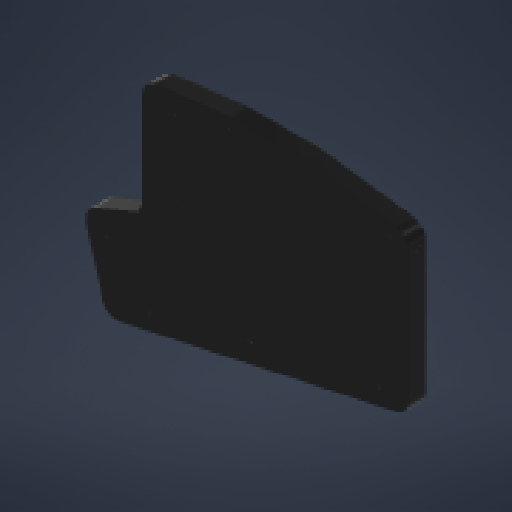
# Autodesk Inventor part: Case Bottom
Saved by Autodesk Inventor 2024.3 (Build 283343000, 343)
## iProperties
Created: 2024-12-13
Part Number: Case Bottom
Material: Generic
Document SubType Name: Modeling
Designer: micha
Density: 1 g/cm^3
Appearance: Smooth - Black
Author: micha
Autodesk Inventor part; units mm, degrees
ref_plane "YZ Plane" through (0, 0, 0) normal (1, 0, 0) x (0, 1, 0)
ref_plane "XZ Plane" through (0, 0, 0) normal (0, 1, 0) x (-1, 0, 0)
ref_plane "XY Plane" through (0, 0, 0) normal (0, 0, 1) x (1, 0, 0)
sketch "Sketch1" plane through (0, 0, 0) normal (0, 0, 1) x (1, 0, 0)
  arc A0 (-212.538998, -59.46938) -> (-218.504473, -64.85881) centre (-212.540124, -65.464394) ccw
  line L0 (-174.03635, -54.760868) -> (-212.538998, -59.46938)
  arc A1 (-171.723941, -54.62) -> (-174.03635, -54.760868) centre (-171.723929, -73.670234) ccw
  line L1 (-134.883154, -54.62) -> (-171.723941, -54.62)
  arc A2 (-132.280238, -54.798664) -> (-134.883154, -54.62) centre (-134.883228, -73.671057) ccw
  line L2 (-83.542158, -61.521089) -> (-132.280238, -54.798664)
  arc A3 (-79.229999, -66.473551) -> (-83.542158, -61.521089) centre (-84.229999, -66.47355) ccw
  line L3 (-79.477279, -138.022361) -> (-79.229999, -66.473551)
  arc A4 (-82.987736, -142.795333) -> (-79.477279, -138.022361) centre (-84.477328, -138.022325) ccw
  line L4 (-234.360737, -175.723727) -> (-82.987736, -142.795333)
  arc A5 (-240.233758, -172.877296) -> (-234.360737, -175.723727) centre (-235.745406, -171.098608) ccw
  line L5 (-249.32837, -140.9769) -> (-240.233758, -172.877296)
  arc A6 (-246.255809, -134.396385) -> (-249.32837, -140.9769) centre (-243.556977, -139.664093) ccw
  line L6 (-224.253241, -125.409604) -> (-246.255809, -134.396385)
  arc A7 (-224.253241, -125.409604) -> (-221.422813, -123.130228) centre (-226.654291, -119.531049) ccw
  line L7 (-220.681757, -122.053089) -> (-221.422813, -123.130228)
  arc A8 (-220.681757, -122.053089) -> (-218.444728, -114.839545) centre (-231.14451, -114.854791) ccw
  line L8 (-218.504474, -64.85881) -> (-218.444728, -114.839545)
  circle A9 centre (-163.195, -152.4) radius 1.05
  circle A10 centre (-92.075, -138.43) radius 1.05
  circle A11 centre (-86.11, -127.04) radius 0.8509
  circle A12 centre (-91.61, -127.04) radius 1.7145
  circle A13 centre (-97.11, -127.04) radius 0.8509
  circle A14 centre (-104.11, -127.04) radius 0.8509
  circle A15 centre (-122.11, -139.04) radius 0.8509
  circle A16 centre (-122.61, -135.29) radius 1.5
  circle A17 centre (-109.61, -127.04) radius 1.7145
  circle A18 centre (-115.11, -127.04) radius 0.8509
  circle A19 centre (-86.61, -123.29) radius 1.5
  circle A20 centre (-91.61, -121.09) radius 1.5
  circle A21 centre (-96.61, -123.29) radius 1.5
  circle A22 centre (-104.61, -123.29) radius 1.5
  circle A23 centre (-109.61, -121.09) radius 1.5
  circle A24 centre (-114.61, -123.29) radius 1.5
  circle A25 centre (-122.11, -122.04) radius 0.8509
  circle A26 centre (-122.61, -118.29) radius 1.5
  circle A27 centre (-127.61, -139.04) radius 1.7145
  circle A28 centre (-133.11, -139.04) radius 0.8509
  circle A29 centre (-132.61, -135.29) radius 1.5
  circle A30 centre (-140.11, -136.54) radius 0.8509
  circle A31 centre (-127.61, -133.09) radius 1.5
  circle A32 centre (-140.61, -132.79) radius 1.5
  circle A33 centre (-145.61, -136.54) radius 1.7145
  circle A34 centre (-151.11, -136.54) radius 0.8509
  circle A35 centre (-158.11, -139.04) radius 0.8509
  circle A36 centre (-163.61, -139.04) radius 1.7145
  circle A37 centre (-158.61, -135.29) radius 1.5
  circle A38 centre (-145.61, -130.59) radius 1.5
  circle A39 centre (-150.61, -132.79) radius 1.5
  circle A40 centre (-163.61, -133.09) radius 1.5
  circle A41 centre (-127.61, -122.04) radius 1.7145
  circle A42 centre (-133.11, -122.04) radius 0.8509
  circle A43 centre (-140.11, -119.54) radius 0.8509
  circle A44 centre (-127.61, -116.09) radius 1.5
  circle A45 centre (-132.61, -118.29) radius 1.5
  circle A46 centre (-140.61, -115.79) radius 1.5
  circle A47 centre (-145.61, -119.54) radius 1.7145
  circle A48 centre (-151.11, -119.54) radius 0.8509
  circle A49 centre (-158.11, -122.04) radius 0.8509
  circle A50 centre (-163.61, -122.04) radius 1.7145
  circle A51 centre (-145.61, -113.59) radius 1.5
  circle A52 centre (-150.61, -115.79) radius 1.5
  circle A53 centre (-158.61, -118.29) radius 1.5
  circle A54 centre (-163.61, -116.09) radius 1.5
  circle A55 centre (-198.250758, -148.049295) radius 0.8509
  circle A56 centre (-187.91414, -144.287073) radius 0.8509
  circle A57 centre (-193.082449, -146.168184) radius 1.7145
  circle A58 centre (-189.666561, -140.934236) radius 1.5
  circle A59 centre (-199.063488, -144.354437) radius 1.5
  circle A60 centre (-195.117469, -140.577013) radius 1.5
  circle A61 centre (-217.896589, -166.960904) radius 1.05
  circle A62 centre (-217.279534, -154.975203) radius 0.8509
  circle A63 centre (-236.308309, -161.901111) radius 0.8509
  circle A64 centre (-225.971691, -158.138889) radius 0.8509
  circle A65 centre (-231.14, -160.02) radius 1.7145
  circle A66 centre (-227.724112, -154.786052) radius 1.5
  circle A67 centre (-237.121039, -158.206253) radius 1.5
  circle A68 centre (-233.17502, -154.428829) radius 1.5
  circle A69 centre (-206.942916, -151.212981) radius 0.8509
  circle A70 centre (-212.111225, -153.094092) radius 1.7145
  circle A71 centre (-208.695337, -147.860144) radius 1.5
  circle A72 centre (-218.092264, -151.280345) radius 1.5
  circle A73 centre (-214.146245, -147.502921) radius 1.5
  circle A74 centre (-241.3, -142.24) radius 1.05
  circle A75 centre (-169.11, -139.04) radius 0.8509
  circle A76 centre (-168.61, -135.29) radius 1.5
  circle A77 centre (-201.862915, -128.352981) radius 0.8509
  circle A78 centre (-169.11, -122.04) radius 0.8509
  circle A79 centre (-176.11, -124.54) radius 0.8509
  circle A80 centre (-181.61, -124.54) radius 1.7145
  circle A81 centre (-176.61, -120.79) radius 1.5
  circle A82 centre (-168.61, -118.29) radius 1.5
  circle A83 centre (-181.61, -118.59) radius 1.5
  circle A84 centre (-187.11, -124.54) radius 0.8509
  circle A85 centre (-186.61, -120.79) radius 1.5
  circle A86 centre (-194.500629, -125.059163) radius 0.4
  circle A87 centre (-194.500629, -123.059163) radius 0.381
  circle A88 centre (-194.500629, -121.059163) radius 0.381
  circle A89 centre (-201.350629, -114.209163) radius 0.4
  circle A90 centre (-220.891691, -135.278889) radius 0.8509
  circle A91 centre (-207.031224, -130.234092) radius 1.7145
  circle A92 centre (-212.199533, -132.115203) radius 0.8509
  circle A93 centre (-222.644112, -131.926052) radius 1.5
  circle A94 centre (-213.012263, -128.420345) radius 1.5
  circle A95 centre (-226.06, -137.16) radius 1.7145
  circle A96 centre (-231.228309, -139.041111) radius 0.8509
  circle A97 centre (-232.041039, -135.346253) radius 1.5
  circle A98 centre (-228.09502, -131.568829) radius 1.5
  circle A99 centre (-203.615336, -125.000144) radius 1.5
  circle A100 centre (-209.066244, -124.642921) radius 1.5
  circle A101 centre (-203.350629, -114.209163) radius 0.4
  circle A102 centre (-205.350629, -114.209163) radius 0.4
  circle A103 centre (-86.11, -110.04) radius 0.8509
  circle A104 centre (-91.61, -110.04) radius 1.7145
  circle A105 centre (-86.61, -106.29) radius 1.5
  circle A106 centre (-97.11, -110.04) radius 0.8509
  circle A107 centre (-104.11, -110.04) radius 0.8509
  circle A108 centre (-96.61, -106.29) radius 1.5
  circle A109 centre (-104.61, -106.29) radius 1.5
  circle A110 centre (-91.61, -104.09) radius 1.5
  circle A111 centre (-109.61, -110.04) radius 1.7145
  circle A112 centre (-115.11, -110.04) radius 0.8509
  circle A113 centre (-114.61, -106.29) radius 1.5
  circle A114 centre (-109.61, -104.09) radius 1.5
  circle A115 centre (-122.11, -105.04) radius 0.8509
  circle A116 centre (-122.61, -101.29) radius 1.5
  circle A117 centre (-86.11, -93.04) radius 0.8509
  circle A118 centre (-91.61, -93.04) radius 1.7145
  circle A119 centre (-97.11, -93.04) radius 0.8509
  circle A120 centre (-104.11, -93.04) radius 0.8509
  circle A121 centre (-86.61, -89.29) radius 1.5
  circle A122 centre (-91.61, -87.09) radius 1.5
  circle A123 centre (-96.61, -89.29) radius 1.5
  circle A124 centre (-104.61, -89.29) radius 1.5
  circle A125 centre (-109.61, -93.04) radius 1.7145
  circle A126 centre (-115.11, -93.04) radius 0.8509
  circle A127 centre (-109.61, -87.09) radius 1.5
  circle A128 centre (-114.61, -89.29) radius 1.5
  circle A129 centre (-122.11, -88.04) radius 0.8509
  circle A130 centre (-127.61, -105.04) radius 1.7145
  circle A131 centre (-133.11, -105.04) radius 0.8509
  circle A132 centre (-127.61, -99.09) radius 1.5
  circle A133 centre (-132.61, -101.29) radius 1.5
  circle A134 centre (-140.11, -102.54) radius 0.8509
  circle A135 centre (-140.61, -98.79) radius 1.5
  circle A136 centre (-145.61, -102.54) radius 1.7145
  circle A137 centre (-151.11, -102.54) radius 0.8509
  circle A138 centre (-150.61, -98.79) radius 1.5
  circle A139 centre (-158.11, -105.04) radius 0.8509
  circle A140 centre (-163.61, -105.04) radius 1.7145
  circle A141 centre (-158.61, -101.29) radius 1.5
  circle A142 centre (-163.61, -99.09) radius 1.5
  circle A143 centre (-127.61, -88.04) radius 1.7145
  circle A144 centre (-133.11, -88.04) radius 0.8509
  circle A145 centre (-140.11, -85.54) radius 0.8509
  circle A146 centre (-145.61, -96.59) radius 1.5
  circle A147 centre (-145.61, -85.54) radius 1.7145
  circle A148 centre (-151.11, -85.54) radius 0.8509
  circle A149 centre (-158.11, -88.04) radius 0.8509
  circle A150 centre (-163.61, -88.04) radius 1.7145
  circle A151 centre (-86.11, -76.04) radius 0.8509
  circle A152 centre (-91.61, -76.04) radius 1.7145
  circle A153 centre (-86.61, -72.29) radius 1.5
  circle A154 centre (-97.11, -76.04) radius 0.8509
  circle A155 centre (-104.11, -76.04) radius 0.8509
  circle A156 centre (-96.61, -72.29) radius 1.5
  circle A157 centre (-104.61, -72.29) radius 1.5
  circle A158 centre (-122.61, -84.29) radius 1.5
  circle A159 centre (-109.61, -76.04) radius 1.7145
  circle A160 centre (-115.11, -76.04) radius 0.8509
  circle A161 centre (-114.61, -72.29) radius 1.5
  circle A162 centre (-122.11, -71.04) radius 0.8509
  circle A163 centre (-91.61, -70.09) radius 1.5
  circle A164 centre (-86.119409, -65.103368) radius 1.05
  circle A165 centre (-109.61, -70.09) radius 1.5
  circle A166 centre (-122.61, -67.29) radius 1.5
  circle A167 centre (-127.61, -82.09) radius 1.5
  circle A168 centre (-132.61, -84.29) radius 1.5
  circle A169 centre (-140.61, -81.79) radius 1.5
  circle A170 centre (-127.61, -71.04) radius 1.7145
  circle A171 centre (-133.11, -71.04) radius 0.8509
  circle A172 centre (-150.61, -81.79) radius 1.5
  circle A173 centre (-145.61, -79.59) radius 1.5
  circle A174 centre (-158.61, -84.29) radius 1.5
  circle A175 centre (-163.61, -82.09) radius 1.5
  circle A176 centre (-158.11, -71.04) radius 0.8509
  circle A177 centre (-163.61, -71.04) radius 1.7145
  circle A178 centre (-127.61, -65.09) radius 1.5
  circle A179 centre (-132.61, -67.29) radius 1.5
  circle A180 centre (-140.11, -68.54) radius 0.8509
  circle A181 centre (-140.61, -64.79) radius 1.5
  circle A182 centre (-145.61, -68.54) radius 1.7145
  circle A183 centre (-151.11, -68.54) radius 0.8509
  circle A184 centre (-150.61, -64.79) radius 1.5
  circle A185 centre (-158.61, -67.29) radius 1.5
  circle A186 centre (-163.61, -65.09) radius 1.5
  circle A187 centre (-145.61, -62.59) radius 1.5
  circle A188 centre (-176.11, -107.54) radius 0.8509
  circle A189 centre (-181.61, -107.54) radius 1.7145
  circle A190 centre (-169.11, -105.04) radius 0.8509
  circle A191 centre (-168.61, -101.29) radius 1.5
  circle A192 centre (-176.61, -103.79) radius 1.5
  circle A193 centre (-181.61, -101.59) radius 1.5
  circle A194 centre (-187.11, -107.54) radius 0.8509
  circle A195 centre (-202.046541, -105.604357) radius 1.05
  circle A196 centre (-186.61, -103.79) radius 1.5
  circle A197 centre (-169.11, -88.04) radius 0.8509
  circle A198 centre (-176.11, -90.54) radius 0.8509
  circle A199 centre (-181.61, -90.54) radius 1.7145
  circle A200 centre (-176.61, -86.79) radius 1.5
  circle A201 centre (-195.58, -92.956268) radius 0.5461
  circle A202 centre (-187.11, -90.54) radius 0.8509
  circle A203 centre (-186.61, -86.79) radius 1.5
  circle A204 centre (-195.58, -90.416268) radius 0.5461
  circle A205 centre (-195.58, -87.876268) radius 0.5461
  circle A206 centre (-195.58, -85.336268) radius 0.5461
  arc A207 (-207.555848, -104.429405) -> (-207.555848, -103.529405) centre (-207.555848, -103.979405) ccw
  line L9 (-207.555848, -103.529405) -> (-208.155848, -103.529405)
  arc A208 (-208.155848, -103.529405) -> (-208.155848, -104.429405) centre (-208.155848, -103.979405) ccw
  line L10 (-208.155848, -104.429405) -> (-207.555848, -104.429405)
  arc A209 (-211.555848, -104.429405) -> (-211.555848, -103.529405) centre (-211.555848, -103.979405) ccw
  line L11 (-211.555848, -103.529405) -> (-212.155848, -103.529405)
  arc A210 (-212.155848, -103.529405) -> (-212.155848, -104.429405) centre (-212.155848, -103.979405) ccw
  line L12 (-212.155848, -104.429405) -> (-211.555848, -104.429405)
  arc A211 (-206.455848, -102.129405) -> (-206.455848, -101.229405) centre (-206.455848, -101.679405) ccw
  line L13 (-206.455848, -101.229405) -> (-207.055848, -101.229405)
  arc A212 (-207.055848, -101.229405) -> (-207.055848, -102.129405) centre (-207.055848, -101.679405) ccw
  line L14 (-207.055848, -102.129405) -> (-206.455848, -102.129405)
  arc A213 (-206.455848, -99.829405) -> (-206.455848, -98.929405) centre (-206.455848, -99.379405) ccw
  line L15 (-206.455848, -98.929405) -> (-207.055848, -98.929405)
  arc A214 (-207.055848, -98.929405) -> (-207.055848, -99.829405) centre (-207.055848, -99.379405) ccw
  line L16 (-207.055848, -99.829405) -> (-206.455848, -99.829405)
  circle A215 centre (-209.455848, -101.679405) radius 0.75
  circle A216 centre (-209.455848, -99.379405) radius 0.75
  arc A217 (-214.555848, -104.429405) -> (-214.555848, -103.529405) centre (-214.555848, -103.979405) ccw
  line L17 (-214.555848, -103.529405) -> (-215.155848, -103.529405)
  arc A218 (-215.155848, -103.529405) -> (-215.155848, -104.429405) centre (-215.155848, -103.979405) ccw
  line L18 (-215.155848, -104.429405) -> (-214.555848, -104.429405)
  circle A219 centre (-216.455848, -101.679405) radius 0.75
  circle A220 centre (-216.455848, -99.379405) radius 0.75
  arc A221 (-207.555848, -97.529405) -> (-207.555848, -96.629405) centre (-207.555848, -97.079405) ccw
  line L19 (-207.555848, -96.629405) -> (-208.155848, -96.629405)
  arc A222 (-208.155848, -96.629405) -> (-208.155848, -97.529405) centre (-208.155848, -97.079405) ccw
  line L20 (-208.155848, -97.529405) -> (-207.555848, -97.529405)
  arc A223 (-211.555848, -97.529405) -> (-211.555848, -96.629405) centre (-211.555848, -97.079405) ccw
  line L21 (-211.555848, -96.629405) -> (-212.155848, -96.629405)
  arc A224 (-212.155848, -96.629405) -> (-212.155848, -97.529405) centre (-212.155848, -97.079405) ccw
  line L22 (-212.155848, -97.529405) -> (-211.555848, -97.529405)
  circle A225 centre (-210.82, -92.956268) radius 0.5461
  arc A226 (-214.555848, -97.529405) -> (-214.555848, -96.629405) centre (-214.555848, -97.079405) ccw
  line L23 (-214.555848, -96.629405) -> (-215.155848, -96.629405)
  arc A227 (-215.155848, -96.629405) -> (-215.155848, -97.529405) centre (-215.155848, -97.079405) ccw
  line L24 (-215.155848, -97.529405) -> (-214.555848, -97.529405)
  circle A228 centre (-210.82, -90.416268) radius 0.5461
  circle A229 centre (-210.82, -87.876268) radius 0.5461
  circle A230 centre (-210.82, -85.336268) radius 0.5461
  circle A231 centre (-168.61, -84.29) radius 1.5
  circle A232 centre (-181.61, -84.59) radius 1.5
  circle A233 centre (-169.11, -71.04) radius 0.8509
  circle A234 centre (-176.11, -73.54) radius 0.8509
  circle A235 centre (-181.61, -73.54) radius 1.7145
  circle A236 centre (-195.58, -82.796268) radius 0.5461
  circle A237 centre (-195.58, -80.256268) radius 0.5461
  circle A238 centre (-187.11, -73.54) radius 0.8509
  circle A239 centre (-195.58, -77.716268) radius 0.5461
  circle A240 centre (-195.58, -75.176268) radius 0.5461
  circle A241 centre (-199.5, -77.736268) radius 0.2
  circle A242 centre (-199.45, -75.286268) radius 0.2
  circle A243 centre (-195.58, -72.636268) radius 0.5461
  circle A244 centre (-199.45, -72.636268) radius 0.2
  circle A245 centre (-168.61, -67.29) radius 1.5
  circle A246 centre (-176.61, -69.79) radius 1.5
  circle A247 centre (-181.61, -67.59) radius 1.5
  circle A248 centre (-174.342576, -58.074257) radius 1.05
  circle A249 centre (-186.61, -69.79) radius 1.5
  circle A250 centre (-195.58, -70.096268) radius 0.5461
  circle A251 centre (-195.58, -67.556268) radius 0.5461
  circle A252 centre (-199.486417, -69.986269) radius 0.2
  circle A253 centre (-195.58, -65.016268) radius 0.5461
  circle A254 centre (-210.82, -82.796268) radius 0.5461
  circle A255 centre (-210.82, -80.256268) radius 0.5461
  circle A256 centre (-206.55, -77.786268) radius 0.2
  circle A257 centre (-206.55, -75.236268) radius 0.2
  circle A258 centre (-210.82, -77.716268) radius 0.5461
  circle A259 centre (-210.82, -75.176268) radius 0.5461
  circle A260 centre (-206.55, -72.636268) radius 0.2
  circle A261 centre (-210.82, -72.636268) radius 0.5461
  circle A262 centre (-206.55, -70.186268) radius 0.2
  circle A263 centre (-210.82, -70.096268) radius 0.5461
  circle A264 centre (-210.82, -67.556268) radius 0.5461
  circle A265 centre (-204.203785, -64.736757) radius 1.05
  circle A266 centre (-210.82, -65.016268) radius 0.5461
  arc A267 (-212.752532, -56.29684) -> (-221.663233, -64.538089) centre (-212.540124, -65.464394) ccw
  line L25 (-212.752532, -56.29684) -> (-174.421768, -51.609348)
  arc A268 (-171.723929, -51.445) -> (-174.421768, -51.609348) centre (-171.723929, -73.670234) ccw
  line L26 (-171.723929, -51.445) -> (-134.883228, -51.445)
  arc A269 (-131.846348, -51.653451) -> (-134.883228, -51.445) centre (-134.883228, -73.671057) ccw
  line L27 (-131.846348, -51.653451) -> (-83.113, -58.375223)
  arc A270 (-76.055001, -66.479709) -> (-83.113, -58.375223) centre (-84.229999, -66.47355) ccw
  line L28 (-76.055001, -66.479709) -> (-76.302281, -138.028529)
  arc A271 (-82.192563, -145.87161) -> (-76.302281, -138.028529) centre (-84.477328, -138.022325) ccw
  line L29 (-82.192563, -145.87161) -> (-233.581807, -178.803537)
  arc A272 (-243.249182, -173.880774) -> (-233.581807, -178.803537) centre (-235.745406, -171.098608) ccw
  line L30 (-243.249182, -173.880774) -> (-252.402726, -141.773666)
  arc A273 (-247.568867, -131.503069) -> (-252.402726, -141.773666) centre (-243.556977, -139.664093) ccw
  line L31 (-247.568867, -131.503069) -> (-225.453766, -122.470324)
  arc A274 (-225.453766, -122.470324) -> (-224.038554, -121.330638) centre (-226.654291, -119.531049) ccw
  line L32 (-224.038554, -121.330638) -> (-223.297462, -120.253446)
  arc A275 (-223.297462, -120.253446) -> (-221.619726, -114.843405) centre (-231.14451, -114.854791) ccw
  line L33 (-221.619726, -114.843405) -> (-221.663233, -78.447127)
  line L34 (-221.663233, -78.447127) -> (-221.663233, -64.538089)
  point P0 (0, 0)
  point P1 (-218.504473, -64.85881)
  dimension "d0" = 3.175
  constraints: 20 end point, 18 point on circle, 9 centre point, 1 vertical, 17 other
  measures "d0" distance between parallel lines of L3 L28
extrude "Extrusion1" add sketch "Sketch1" along normal blind 3.175 contours L0 A1 L1 A2 L2 A3 L3 A4 L4 A5 L5 A6 L6 A7 L7 A8 L8 A0 | A11 | A12 | A13 | A14 | A15 | A16 | A17 | A18 | A19 | A20 | A21 | A22 | A23 | A24 | A25 | A26 | A27 | A28 | A29 | A30 | A31 | A32 | A33 | A34 | A35 | A36 | A37 | A38 | A39 | A40 | A41 | A42 | A43 | A44 | A45 | A46 | A47 | A48 | A49 | A50 | A51 | A52 | A53 | A54 | A55 | A56 | A57 | A58 | A59 | A60 | A62 | A63 | A64 | A65 | A66 | A67 | A68 | A69 | A70 | A71 | A72 | A73 | A75 | A76 | A77 | A78 | A79 | A80 | A81 | A82 | A83 | A84 | A85 | A86 | A87 | A88 | A89 | A90 | A91 | A92 | A93 | A94 | A95 | A96 | A97 | A98 | A99 | A100 | A101 | A102 | A103 | A104 | A105 | A106 | A107 | A108 | A109 | A110 | A111 | A112 | A113 | A114 | A115 | A116 | A117 | A118 | A119 | A120 | A121 | A122 | A123 | A124 | A125 | A126 | A127 | A128 | A129 | A130 | A131 | A132 | A133 | A134 | A135 | A136 | A137 | A138 | A139 | A140 | A141 | A142 | A143 | A144 | A145 | A146 | A147 | A148 | A149 | A150 | A151 | A152 | A153 | A154 | A155 | A156 | A157 | A158 | A159 | A160 | A161 | A162 | A163 | A165 | A166 | A167 | A168 | A169 | A170 | A171 | A172 | A173 | A174 | A175 | A176 | A177 | A178 | A179 | A180 | A181 | A182 | A183 | A184 | A185 | A186 | A187 | A188 | A189 | A190 | A191 | A192 | A193 | A194 | A196 | A197 | A198 | A199 | A200 | A201 | A202 | A203 | A204 | A205 | A206 | L10 A208 L9 A207 | L12 A210 L11 A209 | L14 A212 L13 A211 | L16 A214 L15 A213 | A215 | A216 | L18 A218 L17 A217 | A219 | A220 | L20 A222 L19 A221 | L22 A224 L21 A223 | A225 | L24 A227 L23 A226 | A228 | A229 | A230 | A231 | A232 | A233 | A234 | A235 | A236 | A237 | A238 | A239 | A240 | A241 | A242 | A243 | A244 | A245 | A246 | A247 | A249 | A250 | A251 | A252 | A253 | A254 | A255 | A256 | A257 | A258 | A259 | A260 | A261 | A262 | A263 | A264 | A266 | L25 A268 L26 A269 L27 A270 L28 A271 L29 A272 L30 A273 L31 A274 L32 A275 L33 L34 A267
sketch "Sketch2" plane through (0, 0, 0) normal (0, 0, -1) x (-1, 0, 0)
  line L0 (174.421768, -51.609348) -> (212.752532, -56.29684)
  arc A0 (174.421768, -51.609348) -> (171.723929, -51.445) centre (171.723929, -73.670234) ccw
  line L1 (134.883228, -51.445) -> (171.723929, -51.445)
  arc A1 (134.883228, -51.445) -> (131.846348, -51.653451) centre (134.883228, -73.671057) ccw
  line L2 (83.112999, -58.375222) -> (131.846348, -51.653451)
  arc A2 (83.112999, -58.375222) -> (76.055001, -66.479709) centre (84.229999, -66.47355) ccw
  line L3 (76.302281, -138.028529) -> (76.055001, -66.479709)
  arc A3 (76.302281, -138.028529) -> (82.192563, -145.87161) centre (84.477328, -138.022325) ccw
  line L4 (233.581807, -178.803537) -> (82.192563, -145.87161)
  arc A4 (233.581807, -178.803537) -> (243.249182, -173.880774) centre (235.745406, -171.098608) ccw
  line L5 (252.402726, -141.773666) -> (243.249182, -173.880774)
  arc A5 (252.402726, -141.773666) -> (247.568867, -131.503069) centre (243.556977, -139.664093) ccw
  line L6 (225.453766, -122.470324) -> (247.568867, -131.503069)
  arc A6 (224.038554, -121.330638) -> (225.453766, -122.470324) centre (226.654291, -119.531049) ccw
  line L7 (223.297462, -120.253446) -> (224.038554, -121.330638)
  arc A7 (221.619726, -114.843405) -> (223.297462, -120.253446) centre (231.14451, -114.854791) ccw
  line L8 (221.663233, -78.447127) -> (221.619726, -114.843405)
  line L9 (221.663233, -64.538089) -> (221.663233, -78.447127)
  arc A8 (221.663233, -64.538089) -> (212.752532, -56.29684) centre (212.540124, -65.464394) ccw
  line L10 (212.546763, -59.342383) -> (174.051782, -54.634809)
  arc A9 (174.051782, -54.634809) -> (171.723929, -54.493) centre (171.723929, -73.670234) ccw
  line L11 (171.723929, -54.493) -> (134.883228, -54.493)
  arc A10 (134.883228, -54.493) -> (132.262815, -54.672865) centre (134.883228, -73.671057) ccw
  line L12 (132.262815, -54.672865) -> (83.529466, -61.394636)
  arc A11 (83.529466, -61.394636) -> (79.102999, -66.473772) centre (84.229999, -66.47355) ccw
  line L13 (79.102999, -66.473772) -> (79.350279, -138.022582)
  arc A12 (79.350279, -138.022582) -> (82.955292, -142.918245) centre (84.477328, -138.022325) ccw
  line L14 (82.955292, -142.918245) -> (234.329012, -175.846796)
  arc A13 (234.329012, -175.846796) -> (240.354168, -172.918162) centre (235.745406, -171.098608) ccw
  line L15 (240.354168, -172.918162) -> (249.45144, -141.008435)
  arc A14 (249.45144, -141.008435) -> (246.308844, -134.280862) centre (243.556977, -139.664093) ccw
  line L16 (246.308844, -134.280862) -> (224.301261, -125.292032)
  arc A15 (221.527443, -123.058246) -> (224.301261, -125.292032) centre (226.654291, -119.531049) ccw
  line L17 (221.527443, -123.058246) -> (220.786351, -121.981054)
  arc A16 (218.571728, -114.839762) -> (220.786351, -121.981054) centre (231.14451, -114.854791) ccw
  line L18 (218.571728, -114.839762) -> (218.615233, -78.445305)
  line L19 (218.615233, -78.445305) -> (218.615233, -64.708016)
  arc A17 (218.615233, -64.708016) -> (212.546763, -59.342383) centre (212.540124, -65.464394) ccw
  point P0 (0, 0)
  dimension "d3" = 3.048
  constraints: 20 end point, 18 point on circle, 9 centre point, 18 other
  measures "d3" distance between parallel lines of L0 L10
extrude "Extrusion2" add sketch "Sketch2" along normal blind 6.35
sketch "Sketch3" plane through (0, 0, 0) normal (0, 0, -1) x (-1, 0, 0)
  circle A0 centre (131.846348, -59.124257) radius 1.5875
  circle A1 centre (86.119409, -65.103368) radius 1.05
  line L0 (174.421768, -51.609348) -> (212.752532, -56.29684)
  arc A2 (221.663233, -64.538089) -> (212.752532, -56.29684) centre (212.540124, -65.464394) ccw
  line L1 (221.663233, -64.538089) -> (221.663233, -78.447127)
  line L2 (221.663233, -78.447127) -> (221.619726, -114.843405)
  arc A3 (221.619726, -114.843405) -> (223.297462, -120.253446) centre (231.14451, -114.854791) ccw
  line L3 (223.297462, -120.253446) -> (224.038554, -121.330638)
  arc A4 (224.038554, -121.330638) -> (225.453766, -122.470324) centre (226.654291, -119.531049) ccw
  line L4 (225.453766, -122.470324) -> (247.568867, -131.503069)
  arc A5 (252.402726, -141.773666) -> (247.568867, -131.503069) centre (243.556977, -139.664093) ccw
  line L5 (252.402726, -141.773666) -> (243.249182, -173.880774)
  arc A6 (233.581807, -178.803537) -> (243.249182, -173.880774) centre (235.745406, -171.098608) ccw
  line L6 (233.581807, -178.803537) -> (82.192563, -145.87161)
  arc A7 (76.302281, -138.028529) -> (82.192563, -145.87161) centre (84.477328, -138.022325) ccw
  line L7 (76.302281, -138.028529) -> (76.055001, -66.479709)
  arc A8 (83.112999, -58.375222) -> (76.055001, -66.479709) centre (84.229999, -66.47355) ccw
  line L8 (83.112999, -58.375222) -> (131.846348, -51.653451)
  arc A9 (134.883228, -51.445) -> (131.846348, -51.653451) centre (134.883228, -73.671057) ccw
  line L9 (134.883228, -51.445) -> (171.723929, -51.445)
  arc A10 (174.421768, -51.609348) -> (171.723929, -51.445) centre (171.723929, -73.670234) ccw
  circle A11 centre (202.046541, -105.604357) radius 1.05
  circle A12 centre (92.075, -138.43) radius 1.05
  circle A13 centre (86.119409, -65.103368) radius 1.05
  circle A14 centre (204.203785, -64.736757) radius 1.05
  circle A15 centre (174.342576, -58.074257) radius 1.05
  circle A16 centre (241.3, -142.24) radius 1.05
  circle A17 centre (217.896589, -166.960904) radius 1.05
  circle A18 centre (163.195, -152.4) radius 1.05
  circle A19 centre (86.119409, -65.103368) radius 1.84375
  circle A20 centre (92.075, -138.43) radius 1.84375
  circle A21 centre (163.195, -152.4) radius 1.84375
  circle A22 centre (217.896589, -166.960904) radius 1.84375
  circle A23 centre (241.3, -142.24) radius 1.84375
  circle A24 centre (202.046541, -105.604357) radius 1.84375
  circle A25 centre (204.203785, -64.736757) radius 1.84375
  circle A26 centre (174.342576, -58.074257) radius 1.84375
  circle A27 centre (102.078604, -82.67549) radius 1.5875
  circle A28 centre (145.714087, -74.753571) radius 1.5875
  circle A29 centre (177.661494, -81.08799) radius 1.5875
  circle A30 centre (203.153785, -86.052045) radius 1.5875
  circle A31 centre (177.661494, -96.645266) radius 1.5875
  circle A32 centre (145.714087, -90.857143) radius 1.5875
  circle A33 centre (101.818869, -100.207605) radius 1.5875
  circle A34 centre (101.818869, -116.051442) radius 1.5875
  circle A35 centre (145.714087, -108.908728) radius 1.5875
  circle A36 centre (177.661494, -114.463942) radius 1.5875
  circle A37 centre (137.922037, -126.986696) radius 1.5875
  circle A38 centre (171.705076, -130.336869) radius 1.5875
  circle A39 centre (205.253785, -139.6025) radius 1.5875
  circle A40 centre (187.921029, -151.35) radius 1.5875
  circle A41 centre (86.119409, -65.103368) radius 0.9738
  circle A42 centre (174.342576, -58.074257) radius 0.9738
  circle A43 centre (204.203785, -64.736757) radius 0.9738
  circle A44 centre (202.046541, -105.604357) radius 0.9738
  circle A45 centre (241.3, -142.24) radius 0.9738
  circle A46 centre (217.896589, -166.960904) radius 0.9738
  circle A47 centre (163.195, -152.4) radius 0.9738
  circle A48 centre (92.075, -138.43) radius 0.9738
  point P0 (0, 0)
  dimension "d6" = 3.175
  dimension "d7" = 0.79375
  dimension "d8" = 0.79375
  dimension "d9" = 0.79375
  dimension "d10" = 0.79375
  dimension "d11" = 0.79375
  dimension "d12" = 0.79375
  dimension "d13" = 0.79375
  dimension "d14" = 0.79375
  dimension "d15" = 3.175
  dimension "d16" = 3.175
  dimension "d17" = 3.175
  dimension "d18" = 3.175
  dimension "d19" = 3.175
  dimension "d20" = 3.175
  dimension "d21" = 3.175
  dimension "d22" = 3.175
  dimension "d23" = 3.175
  dimension "d24" = 3.175
  dimension "d25" = 3.175
  dimension "d26" = 3.175
  dimension "d27" = 3.175
  dimension "d28" = 3.175
  dimension "d46" = 0.0762
  dimension "d47" = 0.0762
  dimension "d48" = 0.0762
  dimension "d49" = 0.0762
  dimension "d50" = 0.0762
  dimension "d51" = 0.0762
  dimension "d52" = 0.0762
  dimension "d53" = 0.0762
  constraints: 31 centre point
  measures "d6" diameter of A0
  measures "d7" radial gap between concentric circles of A1 A19
  measures "d8" radial gap between concentric circles of A12 A20
  measures "d9" radial gap between concentric circles of A18 A21
  measures "d10" radial gap between concentric circles of A17 A22
  measures "d11" radial gap between concentric circles of A16 A23
  measures "d12" radial gap between concentric circles of A11 A24
  measures "d13" radial gap between concentric circles of A14 A25
  measures "d14" radial gap between concentric circles of A15 A26
  measures "d15" diameter of A27
  measures "d16" diameter of A28
  measures "d17" diameter of A29
  measures "d18" diameter of A30
  measures "d19" diameter of A31
  measures "d20" diameter of A32
  measures "d21" diameter of A33
  measures "d22" diameter of A34
  measures "d23" diameter of A35
  measures "d24" diameter of A36
  measures "d25" diameter of A37
  measures "d26" diameter of A38
  measures "d27" diameter of A39
  measures "d28" diameter of A40
  measures "d46" radial gap between concentric circles of A1 A41
  measures "d47" radial gap between concentric circles of A15 A42
  measures "d48" radial gap between concentric circles of A14 A43
  measures "d49" radial gap between concentric circles of A11 A44
  measures "d50" radial gap between concentric circles of A16 A45
  measures "d51" radial gap between concentric circles of A17 A46
  measures "d52" radial gap between concentric circles of A18 A47
  measures "d53" radial gap between concentric circles of A12 A48
extrude "Extrusion3" add sketch "Sketch3" along normal blind 3.175 and the other way blind 3.175 contours A1 | A11 | A12 | A14 | A15 | A16 | A17 | A18 | A19 | A20 | A21 | A22 | A23 | A24 | A25 | A26 | A27 | A28 | A29 | A30 | A31 | A32 | A33 | A34 | A35 | A36 | A37 | A38 | A39 | A40 | A41 | A42 | A43 | A44 | A45 | A46 | A47 | A48
sketch "Sketch7" plane through (0, 0, -6.35) normal (0, 0, -1) x (-1, 0, 0)
  line L0 (131.846348, -51.653451) -> (83.112999, -58.375222)
  arc A0 (83.112999, -58.375222) -> (76.055001, -66.479709) centre (84.229999, -66.47355) ccw
  line L1 (76.055001, -66.479709) -> (76.302281, -138.028529)
  arc A1 (76.302281, -138.028529) -> (82.192563, -145.87161) centre (84.477328, -138.022325) ccw
  line L2 (82.192563, -145.87161) -> (233.581807, -178.803537)
  arc A2 (233.581807, -178.803537) -> (243.249182, -173.880774) centre (235.745406, -171.098608) ccw
  line L3 (243.249182, -173.880774) -> (252.402726, -141.773666)
  arc A3 (252.402726, -141.773666) -> (247.568867, -131.503069) centre (243.556977, -139.664093) ccw
  line L4 (247.568867, -131.503069) -> (225.453766, -122.470324)
  arc A4 (224.038554, -121.330638) -> (225.453766, -122.470324) centre (226.654291, -119.531049) ccw
  line L5 (224.038554, -121.330638) -> (223.297462, -120.253446)
  arc A5 (221.619726, -114.843405) -> (223.297462, -120.253446) centre (231.14451, -114.854791) ccw
  line L6 (221.619726, -114.843405) -> (221.663233, -78.447127)
  line L7 (221.663233, -78.447127) -> (221.663233, -64.538089)
  arc A6 (221.663233, -64.538089) -> (212.752532, -56.29684) centre (212.540124, -65.464394) ccw
  line L8 (212.752532, -56.29684) -> (174.421768, -51.609348)
  arc A7 (174.421768, -51.609348) -> (171.723929, -51.445) centre (171.723929, -73.670234) ccw
  line L9 (171.723929, -51.445) -> (134.883228, -51.445)
  arc A8 (134.883228, -51.445) -> (131.846348, -51.653451) centre (134.883228, -73.671057) ccw
  arc A9 (218.571728, -114.839762) -> (220.786351, -121.981054) centre (231.14451, -114.854791) ccw
  line L10 (220.786351, -121.981054) -> (221.527443, -123.058246)
  arc A10 (221.527443, -123.058246) -> (224.301261, -125.292032) centre (226.654291, -119.531049) ccw
  line L11 (224.301261, -125.292032) -> (246.308844, -134.280862)
  arc A11 (249.45144, -141.008435) -> (246.308844, -134.280862) centre (243.556977, -139.664093) ccw
  line L12 (249.45144, -141.008435) -> (240.354168, -172.918162)
  arc A12 (234.329012, -175.846796) -> (240.354168, -172.918162) centre (235.745406, -171.098608) ccw
  line L13 (234.329012, -175.846796) -> (82.955292, -142.918245)
  arc A13 (79.350279, -138.022582) -> (82.955292, -142.918245) centre (84.477328, -138.022325) ccw
  line L14 (79.350279, -138.022582) -> (79.102999, -66.473772)
  arc A14 (83.529466, -61.394636) -> (79.102999, -66.473772) centre (84.229999, -66.47355) ccw
  line L15 (83.529466, -61.394636) -> (132.262815, -54.672865)
  arc A15 (134.883228, -54.493) -> (132.262815, -54.672865) centre (134.883228, -73.671057) ccw
  line L16 (134.883228, -54.493) -> (171.723929, -54.493)
  arc A16 (174.051782, -54.634809) -> (171.723929, -54.493) centre (171.723929, -73.670234) ccw
  line L17 (174.051782, -54.634809) -> (212.546763, -59.342383)
  arc A17 (218.615233, -64.708016) -> (212.546763, -59.342383) centre (212.540124, -65.464394) ccw
  line L18 (218.615233, -64.708016) -> (218.615233, -78.445305)
  line L19 (218.615233, -78.445305) -> (218.571728, -114.839762)
  line L20 (132.210757, -54.295438) -> (83.477408, -61.017209)
  arc A18 (83.477408, -61.017209) -> (78.721999, -66.47445) centre (84.229999, -66.47355) ccw
  line L21 (78.721999, -66.47445) -> (78.969279, -138.023262)
  arc A19 (78.969279, -138.023262) -> (82.858353, -143.287069) centre (84.477328, -138.022325) ccw
  line L22 (82.858353, -143.287069) -> (234.234189, -176.216079)
  arc A20 (234.234189, -176.216079) -> (240.715526, -173.040308) centre (235.745406, -171.098608) ccw
  line L23 (240.715526, -173.040308) -> (249.820592, -141.103241)
  arc A21 (249.820592, -141.103241) -> (246.467642, -133.934167) centre (243.556977, -139.664093) ccw
  line L24 (246.467642, -133.934167) -> (224.445324, -124.939319)
  arc A22 (221.841332, -122.842295) -> (224.445324, -124.939319) centre (226.654291, -119.531049) ccw
  line L25 (221.841332, -122.842295) -> (221.10024, -121.765103)
  arc A23 (218.952728, -114.840217) -> (221.10024, -121.765103) centre (231.14451, -114.854791) ccw
  line L26 (218.952728, -114.840217) -> (218.996233, -78.445533)
  line L27 (218.996233, -78.445533) -> (218.996233, -64.684747)
  arc A24 (218.996233, -64.684747) -> (212.570525, -58.961451) centre (212.540124, -65.464394) ccw
  line L28 (212.570525, -58.961451) -> (174.09803, -54.256626)
  arc A25 (174.09803, -54.256626) -> (171.723929, -54.112) centre (171.723929, -73.670234) ccw
  line L29 (171.723929, -54.112) -> (134.883228, -54.112)
  arc A26 (134.883228, -54.112) -> (132.210757, -54.295438) centre (134.883228, -73.671057) ccw
  point P0 (0, 0)
  dimension "d54" = 0.381
  constraints: 20 end point, 18 point on circle, 9 centre point, 18 other
  measures "d54" distance between parallel lines of L15 L20
extrude "Extrusion7" cut sketch "Sketch7" against normal blind 6.35 contours A26 L29 A25 L28 A24 L27 L26 A23 L25 A22 L24 A21 L23 A20 L22 A19 L21 A18 L20
sketch "Sketch8" plane through (0, 0, -6.35) normal (0, 0, -1) x (-1, 0, 0)
  arc A0 (218.996233, -64.684747) -> (212.570525, -58.961451) centre (212.540124, -65.464394) ccw
  line L0 (218.996233, -64.684747) -> (218.996233, -78.445533)
  line L1 (218.996233, -78.445533) -> (218.952728, -114.840217)
  arc A1 (218.952728, -114.840217) -> (221.10024, -121.765103) centre (231.14451, -114.854791) ccw
  line L2 (221.10024, -121.765103) -> (221.841332, -122.842295)
  arc A2 (221.841332, -122.842295) -> (224.445324, -124.939319) centre (226.654291, -119.531049) ccw
  line L3 (224.445324, -124.939319) -> (246.467642, -133.934167)
  arc A3 (249.820592, -141.103241) -> (246.467642, -133.934167) centre (243.556977, -139.664093) ccw
  line L4 (249.820592, -141.103241) -> (240.715526, -173.040308)
  arc A4 (234.234189, -176.216079) -> (240.715526, -173.040308) centre (235.745406, -171.098608) ccw
  line L5 (234.234189, -176.216079) -> (82.858353, -143.287069)
  arc A5 (78.969279, -138.023262) -> (82.858353, -143.287069) centre (84.477328, -138.022325) ccw
  line L6 (78.969279, -138.023262) -> (78.721999, -66.47445)
  arc A6 (83.477408, -61.017209) -> (78.721999, -66.47445) centre (84.229999, -66.47355) ccw
  line L7 (83.477408, -61.017209) -> (132.210757, -54.295438)
  arc A7 (134.883228, -54.112) -> (132.210757, -54.295438) centre (134.883228, -73.671057) ccw
  line L8 (134.883228, -54.112) -> (171.723929, -54.112)
  arc A8 (174.09803, -54.256626) -> (171.723929, -54.112) centre (171.723929, -73.670234) ccw
  line L9 (174.09803, -54.256626) -> (212.570525, -58.961451)
  line L10 (131.846348, -51.653451) -> (83.112999, -58.375222)
  arc A9 (83.112999, -58.375222) -> (76.055001, -66.479709) centre (84.229999, -66.47355) ccw
  line L11 (76.055001, -66.479709) -> (76.302281, -138.028529)
  arc A10 (76.302281, -138.028529) -> (82.192563, -145.87161) centre (84.477328, -138.022325) ccw
  line L12 (82.192563, -145.87161) -> (233.581807, -178.803537)
  arc A11 (233.581807, -178.803537) -> (243.249182, -173.880774) centre (235.745406, -171.098608) ccw
  line L13 (243.249182, -173.880774) -> (252.402726, -141.773666)
  arc A12 (252.402726, -141.773666) -> (247.568867, -131.503069) centre (243.556977, -139.664093) ccw
  line L14 (247.568867, -131.503069) -> (225.453766, -122.470324)
  arc A13 (224.038554, -121.330638) -> (225.453766, -122.470324) centre (226.654291, -119.531049) ccw
  line L15 (224.038554, -121.330638) -> (223.297462, -120.253446)
  arc A14 (221.619726, -114.843405) -> (223.297462, -120.253446) centre (231.14451, -114.854791) ccw
  line L16 (221.619726, -114.843405) -> (221.663233, -78.447127)
  line L17 (221.663233, -78.447127) -> (221.663233, -64.538089)
  arc A15 (221.663233, -64.538089) -> (212.752532, -56.29684) centre (212.540124, -65.464394) ccw
  line L18 (212.752532, -56.29684) -> (174.421768, -51.609348)
  arc A16 (174.421768, -51.609348) -> (171.723929, -51.445) centre (171.723929, -73.670234) ccw
  line L19 (171.723929, -51.445) -> (134.883228, -51.445)
  arc A17 (134.883228, -51.445) -> (131.846348, -51.653451) centre (134.883228, -73.671057) ccw
  line L20 (76.055001, -66.479709) -> (76.055001, -47.429709)
  line L21 (83.112999, -58.375222) -> (83.112999, -47.429709)
  line L22 (83.112999, -47.429709) -> (76.055001, -47.429709)
  line L23 (221.663233, -64.538089) -> (221.663233, -47.429709)
  line L24 (214.602033, -47.429709) -> (221.663233, -47.429709)
  arc A18 (221.663233, -64.538089) -> (212.752532, -56.29684) centre (212.540124, -65.464394) ccw
  line L25 (214.602033, -56.5292) -> (214.602033, -47.429709)
  arc A19 (252.402726, -141.773666) -> (247.568867, -131.503069) centre (243.556977, -139.664093) ccw
  line L26 (252.402726, -141.773666) -> (257.625657, -123.453636)
  line L27 (257.625657, -123.453636) -> (250.913299, -121.261651)
  line L28 (250.913299, -121.261651) -> (247.568867, -131.503069)
  point P0 (0, 0)
  dimension "d59" = 19.05
  dimension "d60" = 7.0612
  dimension "d61" = 0
  dimension "d62" = 19.05
  dimension "d63" = 7.0612
  constraints: 19 end point, 3 perpendicular, 3 vertical, 1 collinear, 1 point on circle
  measures "d59" distance of L11.start L20.end
  measures "d60" distance between parallel lines of L23 L25
  measures "d61" distance between parallel lines of L24 L22
  measures "d62" distance of L13.end L26.end
  measures "d63" distance of L26.end L27.end
sketch "Sketch8 outline for Extrusion8" plane through (0, 0, -6.35) normal (0, 0, -1) x (-1, 0, 0)
  line L0 (250.913299, -121.261651) -> (247.568867, -131.503069)
  line L1 (257.625657, -123.453636) -> (250.913299, -121.261651)
  line L2 (252.402726, -141.773666) -> (257.625657, -123.453636)
  arc A0 (247.568867, -131.503069) -> (252.402726, -141.773666) centre (243.556977, -139.664093) cw
  line L3 (221.663233, -47.429709) -> (214.602033, -47.429709)
  line L4 (221.663233, -64.538089) -> (221.663233, -47.429709)
  arc A1 (214.602033, -56.5292) -> (221.663233, -64.538089) centre (212.540124, -65.464394) cw
  line L5 (214.602033, -47.429709) -> (214.602033, -56.5292)
  line L6 (83.112999, -58.375222) -> (83.112999, -47.429709)
  arc A2 (76.055001, -66.479709) -> (83.112999, -58.375222) centre (84.229998, -66.47355) cw
  line L7 (76.055001, -47.429709) -> (76.055001, -66.479709)
  line L8 (83.112999, -47.429709) -> (76.055001, -47.429709)
extrude "Extrusion8" add sketch "Sketch8 outline for Extrusion8" against normal up to surface (9.525 mm away)
fillet "Fillet1" radius 3.175 10 edges at (-214.602, -56.5292, -1.5875) (-83.113, -58.3752, 1.5875) (-83.113, -58.3752, -3.175) (-247.5689, -131.5031, -1.5875) (-250.9133, -121.2617, -1.5875) (-257.6257, -123.4536, -1.5875) (-221.6632, -47.4297, -1.5875) (-214.602, -47.4297, -1.5875) (-83.113, -47.4297, -1.5875) (-76.055, -47.4297, -1.5875)
sketch "Sketch9" plane through (-221.663233, -78.447127, -6.35) normal (-1, 0, 0) x (0, 0, 1)
  line L0 (0, 27.842418) -> (9.525, 27.842418) construction
  line L1 (0, 0) -> (0, 27.842418) construction
  line L2 (0, 0) -> (9.525, 0) construction
  line L3 (9.525, 0) -> (9.525, 27.842418) construction
  circle A0 centre (4.7625, 25.899318) radius 1.9431
  point P0 (6.35, 78.447127)
  dimension "d67" = 3.8862
  dimension "d68" = 1.9431
  dimension "d69" = 4.7625
  constraints: 1 centre point
  measures "d67" diameter of A0
  measures "d68" distance from line of L0 A0.centre
  measures "d69" distance from line of L3 A0.centre
extrude "Extrusion9" cut sketch "Sketch9" against normal blind 7.62
sketch "Sketch10" plane through (-76.055001, -66.479709, 3.175) normal (1, 0, 0) x (0, 0, -1)
  line L0 (0, 15.875) -> (9.525, 15.875) construction
  line L1 (0, 15.875) -> (0, 0) construction
  line L2 (9.525, 0) -> (0, 0) construction
  line L3 (9.525, 15.875) -> (9.525, 0) construction
  circle A0 centre (4.7625, 13.9319) radius 1.9431
  point P0 (3.175, 66.479709)
  dimension "d72" = 3.8862
  dimension "d73" = 1.9431
  dimension "d74" = 4.7625
  constraints: 1 centre point
  measures "d72" diameter of A0
  measures "d73" distance from line of L0 A0.centre
  measures "d74" distance from line of L1 A0.centre
extrude "Extrusion10" cut sketch "Sketch10" against normal blind 7.62
sketch "Sketch11" plane through (-243.249182, -173.880774, -6.35) normal (-0.9616814, -0.2741696, 0) x (0, 0, 1)
  line L0 (0, 49.379587) -> (9.525, 49.379587) construction
  line L1 (0, 0) -> (0, 49.379587) construction
  line L2 (0, 0) -> (9.525, 0) construction
  line L3 (9.525, 0) -> (9.525, 49.379587) construction
  circle A0 centre (4.7625, 47.436487) radius 1.9431
  point P0 (6.35, 100.526368)
  dimension "d77" = 3.8862
  dimension "d78" = 1.9431
  dimension "d79" = 4.7625
  constraints: 1 centre point
  measures "d77" diameter of A0
  measures "d78" distance from line of L0 A0.centre
  measures "d79" distance from line of L3 A0.centre
extrude "Extrusion11" cut sketch "Sketch11" against normal blind 7.62
sketch "Sketch12" plane through (-221.619726, -114.843405, -6.35) normal (-0.9999993, -0.0011954, 0) x (0, 0, 1)
  line L0 (1.575, 49.980836) -> (1.575, 0.000065)
  line L1 (1.575, 20.933322) -> (-0.0125, 20.933322)
  line L2 (-0.0125, 7.683313) -> (1.575, 7.683313)
  line L3 (-0.0125, 7.683313) -> (-0.0125, 20.933322)
  line L4 (0, 0) -> (0, 36.396305)
  point P0 (6.35, 114.578406)
  point P1 (0, 20.933322)
  point P2 (0, 7.683313)
  constraints: 2 end point, 1 parallel
extrude "Extrusion12" cut sketch "Sketch12" against normal blind 7.62 contours L0 L2 L4 L1
fillet "Fillet2" radius 3.175 4 edges at (-220.3112, -93.9085, -4.775) (-220.3112, -93.9085, -6.35) (-220.2954, -107.1585, -4.775) (-220.2954, -107.1585, -6.35)
equation "\"d8\" = d7"
equation "\"d9\" = d7"
equation "\"d10\" = d7"
equation "\"d11\" = d7"
equation "\"d12\" = d7"
equation "\"d13\" = d7"
equation "\"d14\" = d7"
body "Solid1"
